Autodesk Fusion 360 part; units mm, degrees
note: some values were not read from the file. Chosen so that the rebuilt part matches the saved one: which bodies a step acts on; which face or edge a step refers to. Set by a fixed rule: which sketch regions a step uses.
(part 2 of 3)
  line L303 (277.1753, -95.3023) -> (279.6753, -95.3023)
  line L304 (279.6753, -95.3023) -> (279.6753, -95.8023)
  line L305 (279.6753, -95.8023) -> (277.1753, -95.8023)
  line L306 (274.6753, -80.803) -> (277.1753, -80.803)
  line L307 (279.6753, -80.803) -> (277.1753, -80.803)
  line L308 (279.6753, -81.303) -> (279.6753, -80.803)
  line L309 (274.6753, -81.303) -> (274.6753, -80.803)
  line L310 (277.1753, -81.303) -> (274.6753, -81.303)
  line L311 (277.1753, -81.303) -> (279.6753, -81.303)
  line L312 (260.6253, -95.8023) -> (258.1253, -95.8023)
  line L313 (255.6253, -95.8023) -> (258.1253, -95.8023)
  line L314 (255.6253, -95.3023) -> (255.6253, -95.8023)
  line L315 (260.6253, -95.3023) -> (260.6253, -95.8023)
  line L316 (258.1253, -95.3023) -> (260.6253, -95.3023)
  line L317 (258.1253, -95.3023) -> (255.6253, -95.3023)
  line L318 (258.1253, -81.303) -> (260.6253, -81.303)
  line L319 (260.6253, -81.303) -> (260.6253, -80.803)
  line L320 (260.6253, -80.803) -> (258.1253, -80.803)
  line L321 (255.6253, -80.803) -> (258.1253, -80.803)
  line L322 (255.6253, -81.303) -> (255.6253, -80.803)
  line L323 (258.1253, -81.303) -> (255.6253, -81.303)
  line L324 (239.0753, -81.303) -> (241.5753, -81.303)
  line L325 (236.5753, -80.803) -> (239.0753, -80.803)
  line L326 (236.5753, -81.303) -> (236.5753, -80.803)
  line L327 (241.5753, -95.8023) -> (239.0753, -95.8023)
  line L328 (239.0753, -81.303) -> (236.5753, -81.303)
  line L329 (239.0753, -95.3023) -> (236.5753, -95.3023)
  line L330 (236.5753, -95.3023) -> (236.5753, -95.8023)
  line L331 (241.5753, -81.303) -> (241.5753, -80.803)
  line L332 (241.5753, -80.803) -> (239.0753, -80.803)
  line L333 (241.5753, -95.3023) -> (241.5753, -95.8023)
  line L334 (236.5753, -95.8023) -> (239.0753, -95.8023)
  line L335 (239.0753, -95.3023) -> (241.5753, -95.3023)
  line L336 (217.5253, -95.3023) -> (217.5253, -95.8023)
  line L337 (217.5253, -80.803) -> (220.0253, -80.803)
  line L338 (222.5253, -95.3023) -> (222.5253, -95.8023)
  line L339 (220.0253, -81.303) -> (217.5253, -81.303)
  line L340 (217.5253, -81.303) -> (217.5253, -80.803)
  line L341 (217.5253, -95.8023) -> (220.0253, -95.8023)
  line L342 (220.0253, -95.3023) -> (222.5253, -95.3023)
  line L343 (220.0253, -95.3023) -> (217.5253, -95.3023)
  line L344 (222.5253, -80.803) -> (220.0253, -80.803)
  line L345 (222.5253, -81.303) -> (222.5253, -80.803)
  line L346 (220.0253, -81.303) -> (222.5253, -81.303)
  line L347 (222.5253, -95.8023) -> (220.0253, -95.8023)
  line L348 (198.4753, -95.3023) -> (198.4753, -95.8023)
  line L349 (198.4753, -80.803) -> (200.9753, -80.803)
  line L350 (203.4753, -95.3023) -> (203.4753, -95.8023)
  line L351 (200.9753, -81.303) -> (198.4753, -81.303)
  line L352 (198.4753, -81.303) -> (198.4753, -80.803)
  line L353 (198.4753, -95.8023) -> (200.9753, -95.8023)
  line L354 (200.9753, -95.3023) -> (203.4753, -95.3023)
  line L355 (200.9753, -95.3023) -> (198.4753, -95.3023)
  line L356 (203.4753, -80.803) -> (200.9753, -80.803)
  line L357 (203.4753, -81.303) -> (203.4753, -80.803)
  line L358 (200.9753, -81.303) -> (203.4753, -81.303)
  line L359 (203.4753, -95.8023) -> (200.9753, -95.8023)
  line L360 (179.4253, -95.8023) -> (181.9253, -95.8023)
  line L361 (184.4253, -95.3023) -> (184.4253, -95.8023)
  line L362 (179.4253, -95.3023) -> (179.4253, -95.8023)
  line L363 (181.9253, -95.3023) -> (184.4253, -95.3023)
  line L364 (181.9253, -95.3023) -> (179.4253, -95.3023)
  line L365 (184.4253, -95.8023) -> (181.9253, -95.8023)
  line L366 (179.4253, -81.303) -> (179.4253, -80.803)
  line L367 (179.4253, -80.803) -> (181.9253, -80.803)
  line L368 (184.4253, -81.303) -> (184.4253, -80.803)
  line L369 (181.9253, -81.303) -> (179.4253, -81.303)
  line L370 (181.9253, -81.303) -> (184.4253, -81.303)
  line L371 (184.4253, -80.803) -> (181.9253, -80.803)
  line L372 (160.3753, -95.8023) -> (162.8753, -95.8023)
  line L373 (165.3753, -95.8023) -> (162.8753, -95.8023)
  line L374 (162.8753, -95.3023) -> (165.3753, -95.3023)
  line L375 (165.3753, -95.3023) -> (165.3753, -95.8023)
  line L376 (160.3753, -95.3023) -> (160.3753, -95.8023)
  line L377 (162.8753, -95.3023) -> (160.3753, -95.3023)
  line L378 (160.3753, -81.303) -> (160.3753, -80.803)
  line L379 (165.3753, -81.303) -> (165.3753, -80.803)
  line L380 (162.8753, -81.303) -> (165.3753, -81.303)
  line L381 (160.3753, -80.803) -> (162.8753, -80.803)
  line L382 (165.3753, -80.803) -> (162.8753, -80.803)
  line L383 (162.8753, -81.303) -> (160.3753, -81.303)
  line L384 (141.3253, -95.8023) -> (143.8253, -95.8023)
  line L385 (143.8253, -95.3023) -> (146.3253, -95.3023)
  line L386 (141.3253, -95.3023) -> (141.3253, -95.8023)
  line L387 (146.3253, -95.8023) -> (143.8253, -95.8023)
  line L388 (143.8253, -95.3023) -> (141.3253, -95.3023)
  line L389 (146.3253, -95.3023) -> (146.3253, -95.8023)
  line L390 (141.3253, -81.303) -> (141.3253, -80.803)
  line L391 (143.8253, -81.303) -> (146.3253, -81.303)
  line L392 (143.8253, -81.303) -> (141.3253, -81.303)
  line L393 (146.3253, -81.303) -> (146.3253, -80.803)
  line L394 (141.3253, -80.803) -> (143.8253, -80.803)
  line L395 (146.3253, -80.803) -> (143.8253, -80.803)
  line L396 (122.2753, -95.3023) -> (122.2753, -95.8023)
  line L397 (124.7753, -95.3023) -> (127.2753, -95.3023)
  line L398 (122.2753, -95.8023) -> (124.7753, -95.8023)
  line L399 (124.7753, -95.3023) -> (122.2753, -95.3023)
  line L400 (127.2753, -95.3023) -> (127.2753, -95.8023)
  line L401 (127.2753, -95.8023) -> (124.7753, -95.8023)
  line L402 (122.2753, -81.303) -> (122.2753, -80.803)
  line L403 (127.2753, -81.303) -> (127.2753, -80.803)
  line L404 (122.2753, -80.803) -> (124.7753, -80.803)
  line L405 (124.7753, -81.303) -> (127.2753, -81.303)
  line L406 (124.7753, -81.303) -> (122.2753, -81.303)
  line L407 (127.2753, -80.803) -> (124.7753, -80.803)
  line L408 (108.2253, -95.3023) -> (108.2253, -95.8023)
  line L409 (108.2253, -95.8023) -> (105.7253, -95.8023)
  line L410 (105.7253, -95.3023) -> (103.2253, -95.3023)
  line L411 (103.2253, -95.8023) -> (105.7253, -95.8023)
  line L412 (105.7253, -95.3023) -> (108.2253, -95.3023)
  line L413 (103.2253, -95.3023) -> (103.2253, -95.8023)
  line L414 (103.2253, -80.803) -> (105.7253, -80.803)
  line L415 (105.7253, -81.303) -> (108.2253, -81.303)
  line L416 (108.2253, -80.803) -> (105.7253, -80.803)
  line L417 (105.7253, -81.303) -> (103.2253, -81.303)
  line L418 (108.2253, -81.303) -> (108.2253, -80.803)
  line L419 (103.2253, -81.303) -> (103.2253, -80.803)
  line L420 (89.1753, -95.3023) -> (89.1753, -95.8023)
  line L421 (84.1753, -95.3023) -> (84.1753, -95.8023)
  line L422 (86.6753, -95.3023) -> (89.1753, -95.3023)
  line L423 (84.1753, -95.8023) -> (86.6753, -95.8023)
  line L424 (86.6753, -95.3023) -> (84.1753, -95.3023)
  line L425 (89.1753, -95.8023) -> (86.6753, -95.8023)
  line L426 (89.1753, -81.303) -> (89.1753, -80.803)
  line L427 (86.6753, -81.303) -> (84.1753, -81.303)
  line L428 (84.1753, -81.303) -> (84.1753, -80.803)
  line L429 (84.1753, -80.803) -> (86.6753, -80.803)
  line L430 (89.1753, -80.803) -> (86.6753, -80.803)
  line L431 (86.6753, -81.303) -> (89.1753, -81.303)
  line L432 (70.1253, -95.3023) -> (70.1253, -95.8023)
  line L433 (67.6253, -95.3023) -> (65.1253, -95.3023)
  line L434 (65.1253, -95.8023) -> (67.6253, -95.8023)
  line L435 (67.6253, -95.3023) -> (70.1253, -95.3023)
  line L436 (65.1253, -95.3023) -> (65.1253, -95.8023)
  line L437 (70.1253, -95.8023) -> (67.6253, -95.8023)
  line L438 (65.1253, -80.803) -> (67.6253, -80.803)
  line L439 (70.1253, -80.803) -> (67.6253, -80.803)
  line L440 (67.6253, -81.303) -> (70.1253, -81.303)
  line L441 (65.1253, -81.303) -> (65.1253, -80.803)
  line L442 (70.1253, -81.303) -> (70.1253, -80.803)
  line L443 (67.6253, -81.303) -> (65.1253, -81.303)
  line L444 (51.0753, -95.8023) -> (48.5753, -95.8023)
  line L445 (51.0753, -95.3023) -> (51.0753, -95.8023)
  line L446 (48.5753, -95.3023) -> (46.0753, -95.3023)
  line L447 (46.0753, -95.3023) -> (46.0753, -95.8023)
  line L448 (48.5753, -95.3023) -> (51.0753, -95.3023)
  line L449 (46.0753, -95.8023) -> (48.5753, -95.8023)
  line L450 (46.0753, -81.303) -> (46.0753, -80.803)
  line L451 (48.5753, -81.303) -> (46.0753, -81.303)
  line L452 (48.5753, -81.303) -> (51.0753, -81.303)
  line L453 (51.0753, -80.803) -> (48.5753, -80.803)
  line L454 (51.0753, -81.303) -> (51.0753, -80.803)
  line L455 (46.0753, -80.803) -> (48.5753, -80.803)
  line L456 (32.0253, -95.8023) -> (29.5253, -95.8023)
  line L457 (27.0253, -95.3023) -> (27.0253, -95.8023)
  line L458 (29.5253, -95.3023) -> (32.0253, -95.3023)
  line L459 (29.5253, -95.3023) -> (27.0253, -95.3023)
  line L460 (32.0253, -95.3023) -> (32.0253, -95.8023)
  line L461 (27.0253, -95.8023) -> (29.5253, -95.8023)
  line L462 (32.0253, -81.303) -> (32.0253, -80.803)
  line L463 (27.0253, -81.303) -> (27.0253, -80.803)
  line L464 (27.0253, -80.803) -> (29.5253, -80.803)
  line L465 (32.0253, -80.803) -> (29.5253, -80.803)
  line L466 (29.5253, -81.303) -> (32.0253, -81.303)
  line L467 (29.5253, -81.303) -> (27.0253, -81.303)
  line L468 (10.4753, -95.3023) -> (7.9753, -95.3023)
  line L469 (7.9753, -95.8023) -> (10.4753, -95.8023)
  line L470 (12.9753, -95.3023) -> (12.9753, -95.8023)
  line L471 (12.9753, -95.8023) -> (10.4753, -95.8023)
  line L472 (7.9753, -95.3023) -> (7.9753, -95.8023)
  line L473 (10.4753, -95.3023) -> (12.9753, -95.3023)
  line L474 (12.9753, -80.803) -> (10.4753, -80.803)
  line L475 (10.4753, -81.303) -> (12.9753, -81.303)
  line L476 (7.9753, -81.303) -> (7.9753, -80.803)
  line L477 (10.4753, -81.303) -> (7.9753, -81.303)
  line L478 (12.9753, -81.303) -> (12.9753, -80.803)
  line L479 (7.9753, -80.803) -> (10.4753, -80.803)
  line L480 (296.2253, -76.2523) -> (298.7253, -76.2523)
  line L481 (298.7253, -76.2523) -> (298.7253, -76.7523)
  line L482 (298.7253, -76.7523) -> (296.2253, -76.7523)
  line L483 (296.2253, -76.2523) -> (293.7253, -76.2523)
  line L484 (293.7253, -76.2523) -> (293.7253, -76.7523)
  line L485 (293.7253, -76.7523) -> (296.2253, -76.7523)
  line L486 (274.9128, -76.2523) -> (274.9128, -76.7523)
  line L487 (272.4128, -76.2523) -> (269.9128, -76.2523)
  line L488 (269.9128, -76.7523) -> (272.4128, -76.7523)
  line L489 (274.9128, -76.7523) -> (272.4128, -76.7523)
  line L490 (272.4128, -76.2523) -> (274.9128, -76.2523)
  line L491 (269.9128, -76.2523) -> (269.9128, -76.7523)
  line L492 (251.1003, -76.7523) -> (248.6003, -76.7523)
  line L493 (248.6003, -76.2523) -> (246.1003, -76.2523)
  line L494 (246.1003, -76.2523) -> (246.1003, -76.7523)
  line L495 (251.1003, -76.2523) -> (251.1003, -76.7523)
  line L496 (248.6003, -76.2523) -> (251.1003, -76.2523)
  line L497 (246.1003, -76.7523) -> (248.6003, -76.7523)
  line L498 (227.0503, -76.2523) -> (227.0503, -76.7523)
  line L499 (229.5503, -76.2523) -> (232.0503, -76.2523)
  line L500 (232.0503, -76.2523) -> (232.0503, -76.7523)
  line L501 (227.0503, -76.7523) -> (229.5503, -76.7523)
  line L502 (232.0503, -76.7523) -> (229.5503, -76.7523)
  line L503 (229.5503, -76.2523) -> (227.0503, -76.2523)
  line L504 (210.5003, -76.2523) -> (208.0003, -76.2523)
  line L505 (208.0003, -76.7523) -> (210.5003, -76.7523)
  line L506 (213.0003, -76.7523) -> (210.5003, -76.7523)
  line L507 (213.0003, -76.2523) -> (213.0003, -76.7523)
  line L508 (208.0003, -76.2523) -> (208.0003, -76.7523)
  line L509 (210.5003, -76.2523) -> (213.0003, -76.2523)
  line L510 (191.4503, -76.2523) -> (188.9503, -76.2523)
  line L511 (193.9503, -76.2523) -> (193.9503, -76.7523)
  line L512 (193.9503, -76.7523) -> (191.4503, -76.7523)
  line L513 (191.4503, -76.2523) -> (193.9503, -76.2523)
  line L514 (188.9503, -76.2523) -> (188.9503, -76.7523)
  line L515 (188.9503, -76.7523) -> (191.4503, -76.7523)
  line L516 (169.9003, -76.7523) -> (172.4003, -76.7523)
  line L517 (172.4003, -76.2523) -> (174.9003, -76.2523)
  line L518 (174.9003, -76.7523) -> (172.4003, -76.7523)
  line L519 (172.4003, -76.2523) -> (169.9003, -76.2523)
  line L520 (169.9003, -76.2523) -> (169.9003, -76.7523)
  line L521 (174.9003, -76.2523) -> (174.9003, -76.7523)
  line L522 (153.3503, -76.2523) -> (150.8503, -76.2523)
  line L523 (155.8503, -76.2523) -> (155.8503, -76.7523)
  line L524 (150.8503, -76.2523) -> (150.8503, -76.7523)
  line L525 (155.8503, -76.7523) -> (153.3503, -76.7523)
  line L526 (153.3503, -76.2523) -> (155.8503, -76.2523)
  line L527 (150.8503, -76.7523) -> (153.3503, -76.7523)
  line L528 (134.3003, -76.2523) -> (131.8003, -76.2523)
  line L529 (131.8003, -76.2523) -> (131.8003, -76.7523)
  line L530 (136.8003, -76.2523) -> (136.8003, -76.7523)
  line L531 (131.8003, -76.7523) -> (134.3003, -76.7523)
  line L532 (136.8003, -76.7523) -> (134.3003, -76.7523)
  line L533 (134.3003, -76.2523) -> (136.8003, -76.2523)
  line L534 (117.7503, -76.7523) -> (115.2503, -76.7523)
  line L535 (112.7503, -76.2523) -> (112.7503, -76.7523)
  line L536 (115.2503, -76.2523) -> (117.7503, -76.2523)
  line L537 (117.7503, -76.2523) -> (117.7503, -76.7523)
  line L538 (115.2503, -76.2523) -> (112.7503, -76.2523)
  line L539 (112.7503, -76.7523) -> (115.2503, -76.7523)
  line L540 (93.7003, -76.7523) -> (96.2003, -76.7523)
  line L541 (93.7003, -76.2523) -> (93.7003, -76.7523)
  line L542 (98.7003, -76.7523) -> (96.2003, -76.7523)
  line L543 (98.7003, -76.2523) -> (98.7003, -76.7523)
  line L544 (96.2003, -76.2523) -> (93.7003, -76.2523)
  line L545 (96.2003, -76.2523) -> (98.7003, -76.2523)
  line L546 (77.1503, -76.2523) -> (79.6503, -76.2523)
  line L547 (79.6503, -76.2523) -> (79.6503, -76.7523)
  line L548 (77.1503, -76.2523) -> (74.6503, -76.2523)
  line L549 (79.6503, -76.7523) -> (77.1503, -76.7523)
  line L550 (74.6503, -76.7523) -> (77.1503, -76.7523)
  line L551 (74.6503, -76.2523) -> (74.6503, -76.7523)
  line L552 (58.1003, -76.2523) -> (60.6003, -76.2523)
  line L553 (60.6003, -76.7523) -> (58.1003, -76.7523)
  line L554 (55.6003, -76.7523) -> (58.1003, -76.7523)
  line L555 (60.6003, -76.2523) -> (60.6003, -76.7523)
  line L556 (58.1003, -76.2523) -> (55.6003, -76.2523)
  line L557 (55.6003, -76.2523) -> (55.6003, -76.7523)
  line L558 (41.5503, -76.7523) -> (39.0503, -76.7523)
  line L559 (36.5503, -76.2523) -> (36.5503, -76.7523)
  line L560 (41.5503, -76.2523) -> (41.5503, -76.7523)
  line L561 (36.5503, -76.7523) -> (39.0503, -76.7523)
  line L562 (39.0503, -76.2523) -> (36.5503, -76.2523)
  line L563 (39.0503, -76.2523) -> (41.5503, -76.2523)
  line L564 (15.2378, -76.2523) -> (17.7378, -76.2523)
  line L565 (17.7378, -76.7523) -> (15.2378, -76.7523)
  line L566 (12.7378, -76.2523) -> (12.7378, -76.7523)
  line L567 (12.7378, -76.7523) -> (15.2378, -76.7523)
  line L568 (15.2378, -76.2523) -> (12.7378, -76.2523)
  line L569 (17.7378, -76.2523) -> (17.7378, -76.7523)
  line L570 (298.7253, -62.253) -> (298.7253, -61.753)
  line L571 (293.7253, -61.753) -> (296.2253, -61.753)
  line L572 (296.2253, -62.253) -> (298.7253, -62.253)
  line L573 (296.2253, -62.253) -> (293.7253, -62.253)
  line L574 (293.7253, -62.253) -> (293.7253, -61.753)
  line L575 (298.7253, -61.753) -> (296.2253, -61.753)
  line L576 (274.9128, -61.753) -> (272.4128, -61.753)
  line L577 (272.4128, -62.253) -> (269.9128, -62.253)
  line L578 (269.9128, -62.253) -> (269.9128, -61.753)
  line L579 (269.9128, -61.753) -> (272.4128, -61.753)
  line L580 (272.4128, -62.253) -> (274.9128, -62.253)
  line L581 (274.9128, -62.253) -> (274.9128, -61.753)
  line L582 (251.1003, -62.253) -> (251.1003, -61.753)
  line L583 (246.1003, -61.753) -> (248.6003, -61.753)
  line L584 (246.1003, -62.253) -> (246.1003, -61.753)
  line L585 (248.6003, -62.253) -> (251.1003, -62.253)
  line L586 (248.6003, -62.253) -> (246.1003, -62.253)
  line L587 (251.1003, -61.753) -> (248.6003, -61.753)
  line L588 (229.5503, -62.253) -> (232.0503, -62.253)
  line L589 (232.0503, -62.253) -> (232.0503, -61.753)
  line L590 (232.0503, -61.753) -> (229.5503, -61.753)
  line L591 (227.0503, -61.753) -> (229.5503, -61.753)
  line L592 (229.5503, -62.253) -> (227.0503, -62.253)
  line L593 (227.0503, -62.253) -> (227.0503, -61.753)
  line L594 (208.0003, -61.753) -> (210.5003, -61.753)
  line L595 (210.5003, -62.253) -> (213.0003, -62.253)
  line L596 (213.0003, -61.753) -> (210.5003, -61.753)
  line L597 (208.0003, -62.253) -> (208.0003, -61.753)
  line L598 (213.0003, -62.253) -> (213.0003, -61.753)
  line L599 (210.5003, -62.253) -> (208.0003, -62.253)
  line L600 (188.9503, -62.253) -> (188.9503, -61.753)
  line L601 (188.9503, -61.753) -> (191.4503, -61.753)
  line L602 (191.4503, -62.253) -> (188.9503, -62.253)
  line L603 (191.4503, -62.253) -> (193.9503, -62.253)
  line L604 (193.9503, -61.753) -> (191.4503, -61.753)
  line L605 (193.9503, -62.253) -> (193.9503, -61.753)
  line L606 (174.9003, -62.253) -> (174.9003, -61.753)
  line L607 (174.9003, -61.753) -> (172.4003, -61.753)
  line L608 (172.4003, -62.253) -> (174.9003, -62.253)
  line L609 (169.9003, -61.753) -> (172.4003, -61.753)
  line L610 (172.4003, -62.253) -> (169.9003, -62.253)
  line L611 (169.9003, -62.253) -> (169.9003, -61.753)
  line L612 (153.3503, -62.253) -> (155.8503, -62.253)
  line L613 (155.8503, -62.253) -> (155.8503, -61.753)
  line L614 (153.3503, -62.253) -> (150.8503, -62.253)
  line L615 (155.8503, -61.753) -> (153.3503, -61.753)
  line L616 (150.8503, -61.753) -> (153.3503, -61.753)
  line L617 (150.8503, -62.253) -> (150.8503, -61.753)
  line L618 (134.3003, -62.253) -> (131.8003, -62.253)
  line L619 (134.3003, -62.253) -> (136.8003, -62.253)
  line L620 (131.8003, -61.753) -> (134.3003, -61.753)
  line L621 (136.8003, -62.253) -> (136.8003, -61.753)
  line L622 (136.8003, -61.753) -> (134.3003, -61.753)
  line L623 (131.8003, -62.253) -> (131.8003, -61.753)
  line L624 (117.7503, -61.753) -> (115.2503, -61.753)
  line L625 (112.7503, -62.253) -> (112.7503, -61.753)
  line L626 (112.7503, -61.753) -> (115.2503, -61.753)
  line L627 (115.2503, -62.253) -> (117.7503, -62.253)
  line L628 (117.7503, -62.253) -> (117.7503, -61.753)
  line L629 (115.2503, -62.253) -> (112.7503, -62.253)
  line L630 (98.7003, -61.753) -> (96.2003, -61.753)
  line L631 (96.2003, -62.253) -> (93.7003, -62.253)
  line L632 (93.7003, -61.753) -> (96.2003, -61.753)
  line L633 (93.7003, -62.253) -> (93.7003, -61.753)
  line L634 (96.2003, -62.253) -> (98.7003, -62.253)
  line L635 (98.7003, -62.253) -> (98.7003, -61.753)
  line L636 (77.1503, -62.253) -> (79.6503, -62.253)
  line L637 (74.6503, -62.253) -> (74.6503, -61.753)
  line L638 (77.1503, -62.253) -> (74.6503, -62.253)
  line L639 (79.6503, -61.753) -> (77.1503, -61.753)
  line L640 (74.6503, -61.753) -> (77.1503, -61.753)
  line L641 (79.6503, -62.253) -> (79.6503, -61.753)
  line L642 (55.6003, -61.753) -> (58.1003, -61.753)
  line L643 (58.1003, -62.253) -> (55.6003, -62.253)
  line L644 (60.6003, -62.253) -> (60.6003, -61.753)
  line L645 (55.6003, -62.253) -> (55.6003, -61.753)
  line L646 (58.1003, -62.253) -> (60.6003, -62.253)
  line L647 (60.6003, -61.753) -> (58.1003, -61.753)
  line L648 (39.0503, -62.253) -> (41.5503, -62.253)
  line L649 (39.0503, -62.253) -> (36.5503, -62.253)
  line L650 (36.5503, -61.753) -> (39.0503, -61.753)
  line L651 (41.5503, -62.253) -> (41.5503, -61.753)
  line L652 (41.5503, -61.753) -> (39.0503, -61.753)
  line L653 (36.5503, -62.253) -> (36.5503, -61.753)
  line L654 (17.7378, -62.253) -> (17.7378, -61.753)
  line L655 (17.7378, -61.753) -> (15.2378, -61.753)
  line L656 (12.7378, -61.753) -> (15.2378, -61.753)
  line L657 (15.2378, -62.253) -> (17.7378, -62.253)
  line L658 (15.2378, -62.253) -> (12.7378, -62.253)
  line L659 (12.7378, -62.253) -> (12.7378, -61.753)
  line L660 (296.2253, -43.203) -> (293.7253, -43.203)
  line L661 (293.7253, -42.703) -> (296.2253, -42.703)
  line L662 (293.7253, -43.203) -> (293.7253, -42.703)
  line L663 (298.7253, -42.703) -> (296.2253, -42.703)
  line L664 (298.7253, -43.203) -> (298.7253, -42.703)
  line L665 (296.2253, -43.203) -> (298.7253, -43.203)
  line L666 (296.2253, -57.2023) -> (293.7253, -57.2023)
  line L667 (296.2253, -57.2023) -> (298.7253, -57.2023)
  line L668 (298.7253, -57.2023) -> (298.7253, -57.7023)
  line L669 (293.7253, -57.2023) -> (293.7253, -57.7023)
  line L670 (293.7253, -57.7023) -> (296.2253, -57.7023)
  line L671 (298.7253, -57.7023) -> (296.2253, -57.7023)
  line L672 (265.2683, -57.2023) -> (262.7683, -57.2023)
  line L673 (262.7683, -57.2023) -> (262.7683, -57.7023)
  line L674 (262.7683, -57.7023) -> (265.2683, -57.7023)
  line L675 (265.2683, -57.2023) -> (267.7683, -57.2023)
  line L676 (267.7683, -57.2023) -> (267.7683, -57.7023)
  line L677 (267.7683, -57.7023) -> (265.2683, -57.7023)
  line L678 (265.2683, -43.203) -> (262.7683, -43.203)
  line L679 (265.2683, -43.203) -> (267.7683, -43.203)
  line L680 (262.7683, -43.203) -> (262.7683, -42.703)
  line L681 (267.7683, -42.703) -> (265.2683, -42.703)
  line L682 (267.7683, -43.203) -> (267.7683, -42.703)
  line L683 (262.7683, -42.703) -> (265.2683, -42.703)
  line L684 (234.3128, -57.2023) -> (231.8128, -57.2023)
  line L685 (231.8128, -57.2023) -> (231.8128, -57.7023)
  line L686 (231.8128, -57.7023) -> (234.3128, -57.7023)
  line L687 (234.3128, -57.2023) -> (236.8128, -57.2023)
  line L688 (236.8128, -57.2023) -> (236.8128, -57.7023)
  line L689 (236.8128, -57.7023) -> (234.3128, -57.7023)
  line L690 (234.3128, -43.203) -> (236.8128, -43.203)
  line L691 (231.8128, -42.703) -> (234.3128, -42.703)
  line L692 (236.8128, -42.703) -> (234.3128, -42.703)
  line L693 (236.8128, -43.203) -> (236.8128, -42.703)
  line L694 (231.8128, -43.203) -> (231.8128, -42.703)
  line L695 (234.3128, -43.203) -> (231.8128, -43.203)
  line L696 (217.7628, -57.7023) -> (215.2628, -57.7023)
  line L697 (215.2628, -57.2023) -> (217.7628, -57.2023)
  line L698 (215.2628, -43.203) -> (217.7628, -43.203)
  line L699 (217.7628, -42.703) -> (215.2628, -42.703)
  line L700 (212.7628, -42.703) -> (215.2628, -42.703)
  line L701 (215.2628, -57.2023) -> (212.7628, -57.2023)
  line L702 (212.7628, -57.2023) -> (212.7628, -57.7023)
  line L703 (212.7628, -43.203) -> (212.7628, -42.703)
  line L704 (217.7628, -57.2023) -> (217.7628, -57.7023)
  line L705 (212.7628, -57.7023) -> (215.2628, -57.7023)
  line L706 (215.2628, -43.203) -> (212.7628, -43.203)
  line L707 (217.7628, -43.203) -> (217.7628, -42.703)
  line L708 (196.2128, -43.203) -> (193.7128, -43.203)
  line L709 (196.2128, -57.2023) -> (193.7128, -57.2023)
  line L710 (193.7128, -57.2023) -> (193.7128, -57.7023)
  line L711 (193.7128, -42.703) -> (196.2128, -42.703)
  line L712 (198.7128, -42.703) -> (196.2128, -42.703)
  line L713 (196.2128, -57.2023) -> (198.7128, -57.2023)
  line L714 (198.7128, -57.7023) -> (196.2128, -57.7023)
  line L715 (198.7128, -43.203) -> (198.7128, -42.703)
  line L716 (196.2128, -43.203) -> (198.7128, -43.203)
  line L717 (198.7128, -57.2023) -> (198.7128, -57.7023)
  line L718 (193.7128, -57.7023) -> (196.2128, -57.7023)
  line L719 (193.7128, -43.203) -> (193.7128, -42.703)
  line L720 (177.1628, -43.203) -> (174.6628, -43.203)
  line L721 (179.6628, -57.2023) -> (179.6628, -57.7023)
  line L722 (174.6628, -57.7023) -> (177.1628, -57.7023)
  line L723 (179.6628, -42.703) -> (177.1628, -42.703)
  line L724 (177.1628, -43.203) -> (179.6628, -43.203)
  line L725 (177.1628, -57.2023) -> (174.6628, -57.2023)
  line L726 (174.6628, -57.2023) -> (174.6628, -57.7023)
  line L727 (174.6628, -42.703) -> (177.1628, -42.703)
  line L728 (179.6628, -57.7023) -> (177.1628, -57.7023)
  line L729 (174.6628, -43.203) -> (174.6628, -42.703)
  line L730 (179.6628, -43.203) -> (179.6628, -42.703)
  line L731 (177.1628, -57.2023) -> (179.6628, -57.2023)
  line L732 (158.1128, -57.2023) -> (155.6128, -57.2023)
  line L733 (160.6128, -57.7023) -> (158.1128, -57.7023)
  line L734 (160.6128, -42.703) -> (158.1128, -42.703)
  line L735 (158.1128, -43.203) -> (160.6128, -43.203)
  line L736 (158.1128, -57.2023) -> (160.6128, -57.2023)
  line L737 (160.6128, -43.203) -> (160.6128, -42.703)
  line L738 (160.6128, -57.2023) -> (160.6128, -57.7023)
  line L739 (155.6128, -42.703) -> (158.1128, -42.703)
  line L740 (155.6128, -57.7023) -> (158.1128, -57.7023)
  line L741 (155.6128, -57.2023) -> (155.6128, -57.7023)
  line L742 (155.6128, -43.203) -> (155.6128, -42.703)
  line L743 (158.1128, -43.203) -> (155.6128, -43.203)
  line L744 (136.5628, -43.203) -> (136.5628, -42.703)
  line L745 (136.5628, -57.7023) -> (139.0628, -57.7023)
  line L746 (136.5628, -42.703) -> (139.0628, -42.703)
  line L747 (141.5628, -42.703) -> (139.0628, -42.703)
  line L748 (139.0628, -57.2023) -> (136.5628, -57.2023)
  line L749 (141.5628, -57.7023) -> (139.0628, -57.7023)
  line L750 (141.5628, -57.2023) -> (141.5628, -57.7023)
  line L751 (139.0628, -57.2023) -> (141.5628, -57.2023)
  line L752 (136.5628, -57.2023) -> (136.5628, -57.7023)
  line L753 (139.0628, -43.203) -> (141.5628, -43.203)
  line L754 (139.0628, -43.203) -> (136.5628, -43.203)
  line L755 (141.5628, -43.203) -> (141.5628, -42.703)
  line L756 (120.0128, -57.2023) -> (117.5128, -57.2023)
  line L757 (117.5128, -57.7023) -> (120.0128, -57.7023)
  line L758 (117.5128, -57.2023) -> (117.5128, -57.7023)
  line L759 (117.5128, -42.703) -> (120.0128, -42.703)
  line L760 (117.5128, -43.203) -> (117.5128, -42.703)
  line L761 (120.0128, -57.2023) -> (122.5128, -57.2023)
  line L762 (120.0128, -43.203) -> (122.5128, -43.203)
  line L763 (122.5128, -57.7023) -> (120.0128, -57.7023)
  line L764 (122.5128, -57.2023) -> (122.5128, -57.7023)
  line L765 (122.5128, -43.203) -> (122.5128, -42.703)
  line L766 (120.0128, -43.203) -> (117.5128, -43.203)
  line L767 (122.5128, -42.703) -> (120.0128, -42.703)
  line L768 (100.9628, -57.2023) -> (103.4628, -57.2023)
  line L769 (103.4628, -57.7023) -> (100.9628, -57.7023)
  line L770 (103.4628, -42.703) -> (100.9628, -42.703)
  line L771 (103.4628, -43.203) -> (103.4628, -42.703)
  line L772 (100.9628, -43.203) -> (103.4628, -43.203)
  line L773 (98.4628, -42.703) -> (100.9628, -42.703)
  line L774 (103.4628, -57.2023) -> (103.4628, -57.7023)
  line L775 (98.4628, -57.7023) -> (100.9628, -57.7023)
  line L776 (100.9628, -57.2023) -> (98.4628, -57.2023)
  line L777 (98.4628, -43.203) -> (98.4628, -42.703)
  line L778 (98.4628, -57.2023) -> (98.4628, -57.7023)
  line L779 (100.9628, -43.203) -> (98.4628, -43.203)
  line L780 (79.4128, -42.703) -> (81.9128, -42.703)
  line L781 (84.4128, -42.703) -> (81.9128, -42.703)
  line L782 (81.9128, -57.2023) -> (79.4128, -57.2023)
  line L783 (79.4128, -57.7023) -> (81.9128, -57.7023)
  line L784 (79.4128, -43.203) -> (79.4128, -42.703)
  line L785 (81.9128, -43.203) -> (84.4128, -43.203)
  line L786 (84.4128, -43.203) -> (84.4128, -42.703)
  line L787 (84.4128, -57.2023) -> (84.4128, -57.7023)
  line L788 (81.9128, -57.2023) -> (84.4128, -57.2023)
  line L789 (79.4128, -57.2023) -> (79.4128, -57.7023)
  line L790 (81.9128, -43.203) -> (79.4128, -43.203)
  line L791 (84.4128, -57.7023) -> (81.9128, -57.7023)
  line L792 (62.8628, -57.2023) -> (60.3628, -57.2023)
  line L793 (65.3628, -57.7023) -> (62.8628, -57.7023)
  line L794 (62.8628, -43.203) -> (60.3628, -43.203)
  line L795 (62.8628, -57.2023) -> (65.3628, -57.2023)
  line L796 (60.3628, -57.7023) -> (62.8628, -57.7023)
  line L797 (65.3628, -42.703) -> (62.8628, -42.703)
  line L798 (62.8628, -43.203) -> (65.3628, -43.203)
  line L799 (60.3628, -42.703) -> (62.8628, -42.703)
  line L800 (65.3628, -43.203) -> (65.3628, -42.703)
  line L801 (60.3628, -57.2023) -> (60.3628, -57.7023)
  line L802 (60.3628, -43.203) -> (60.3628, -42.703)
  line L803 (65.3628, -57.2023) -> (65.3628, -57.7023)
  line L804 (41.3128, -42.703) -> (43.8128, -42.703)
  line L805 (43.8128, -43.203) -> (41.3128, -43.203)
  line L806 (46.3128, -43.203) -> (46.3128, -42.703)
  line L807 (46.3128, -57.2023) -> (46.3128, -57.7023)
  line L808 (41.3128, -43.203) -> (41.3128, -42.703)
  line L809 (43.8128, -57.2023) -> (46.3128, -57.2023)
  line L810 (41.3128, -57.7023) -> (43.8128, -57.7023)
  line L811 (41.3128, -57.2023) -> (41.3128, -57.7023)
  line L812 (46.3128, -57.7023) -> (43.8128, -57.7023)
  line L813 (43.8128, -57.2023) -> (41.3128, -57.2023)
  line L814 (46.3128, -42.703) -> (43.8128, -42.703)
  line L815 (43.8128, -43.203) -> (46.3128, -43.203)
  line L816 (17.6182, -57.2023) -> (15.1182, -57.2023)
  line L817 (15.1182, -57.2023) -> (15.1182, -57.7023)
  line L818 (15.1182, -57.7023) -> (17.6182, -57.7023)
  line L819 (17.6182, -57.2023) -> (20.1182, -57.2023)
  line L820 (20.1182, -57.2023) -> (20.1182, -57.7023)
  line L821 (20.1182, -57.7023) -> (17.6182, -57.7023)
  line L822 (20.1182, -42.703) -> (17.6182, -42.703)
  line L823 (17.6182, -43.203) -> (15.1182, -43.203)
  line L824 (17.6182, -43.203) -> (20.1182, -43.203)
  line L825 (15.1182, -42.703) -> (17.6182, -42.703)
  line L826 (15.1182, -43.203) -> (15.1182, -42.703)
  line L827 (20.1182, -43.203) -> (20.1182, -42.703)
  line L828 (293.7253, -24.1529) -> (293.7253, -23.6529)
  line L829 (293.7253, -23.6529) -> (296.2253, -23.6529)
  line L830 (296.2253, -24.1529) -> (298.7253, -24.1529)
  line L831 (298.7253, -24.1529) -> (298.7253, -23.6529)
  line L832 (296.2253, -24.1529) -> (293.7253, -24.1529)
  line L833 (293.7253, -38.6522) -> (296.2253, -38.6522)
  line L834 (296.2253, -38.1522) -> (298.7253, -38.1522)
  line L835 (296.2253, -38.1522) -> (293.7253, -38.1522)
  line L836 (298.7253, -38.6522) -> (296.2253, -38.6522)
  line L837 (298.7253, -38.1522) -> (298.7253, -38.6522)
  line L838 (298.7253, -23.6529) -> (296.2253, -23.6529)
  line L839 (293.7253, -38.1522) -> (293.7253, -38.6522)
  line L840 (279.6753, -24.1529) -> (279.6753, -23.6529)
  line L841 (279.6753, -38.6522) -> (277.1753, -38.6522)
  line L842 (274.6753, -24.1529) -> (274.6753, -23.6529)
  line L843 (277.1753, -24.1529) -> (279.6753, -24.1529)
  line L844 (274.6753, -38.1522) -> (274.6753, -38.6522)
  line L845 (274.6753, -23.6529) -> (277.1753, -23.6529)
  line L846 (277.1753, -24.1529) -> (274.6753, -24.1529)
  line L847 (274.6753, -38.6522) -> (277.1753, -38.6522)
  line L848 (279.6753, -23.6529) -> (277.1753, -23.6529)
  line L849 (279.6753, -38.1522) -> (279.6753, -38.6522)
  line L850 (277.1753, -38.1522) -> (274.6753, -38.1522)
  line L851 (277.1753, -38.1522) -> (279.6753, -38.1522)
  line L852 (296.2253, -5.1029) -> (293.7253, -5.1029)
  line L853 (293.7253, -19.1022) -> (293.7253, -19.6022)
  line L854 (293.7253, -5.1029) -> (293.7253, -4.6029)
  line L855 (296.2253, -5.1029) -> (298.7253, -5.1029)
  line L856 (296.2253, -19.1022) -> (293.7253, -19.1022)
  line L857 (298.7253, -4.6029) -> (296.2253, -4.6029)
  line L858 (293.7253, -4.6029) -> (296.2253, -4.6029)
  line L859 (298.7253, -19.1022) -> (298.7253, -19.6022)
  line L860 (296.2253, -19.1022) -> (298.7253, -19.1022)
  line L861 (298.7253, -19.6022) -> (296.2253, -19.6022)
  line L862 (298.7253, -5.1029) -> (298.7253, -4.6029)
  line L863 (293.7253, -19.6022) -> (296.2253, -19.6022)
  line L864 (277.1753, -5.1029) -> (279.6753, -5.1029)
  line L865 (274.6753, -19.6022) -> (277.1753, -19.6022)
  line L866 (274.6753, -5.1029) -> (274.6753, -4.6029)
  line L867 (274.6753, -19.1022) -> (274.6753, -19.6022)
  line L868 (274.6753, -4.6029) -> (277.1753, -4.6029)
  line L869 (277.1753, -19.1022) -> (274.6753, -19.1022)
  line L870 (279.6753, -4.6029) -> (277.1753, -4.6029)
  line L871 (279.6753, -5.1029) -> (279.6753, -4.6029)
  line L872 (277.1753, -19.1022) -> (279.6753, -19.1022)
  line L873 (279.6753, -19.6022) -> (277.1753, -19.6022)
  line L874 (277.1753, -5.1029) -> (274.6753, -5.1029)
  line L875 (279.6753, -19.1022) -> (279.6753, -19.6022)
  line L876 (224.7878, -38.1522) -> (222.2878, -38.1522)
  line L877 (222.2878, -38.1522) -> (222.2878, -38.6522)
  line L878 (222.2878, -38.6522) -> (224.7878, -38.6522)
  line L879 (224.7878, -38.1522) -> (227.2878, -38.1522)
  line L880 (227.2878, -38.1522) -> (227.2878, -38.6522)
  line L881 (227.2878, -38.6522) -> (224.7878, -38.6522)
  line L882 (227.2878, -23.6528) -> (224.7878, -23.6528)
  line L883 (222.2878, -24.1528) -> (222.2878, -23.6528)
  line L884 (224.7878, -24.1528) -> (222.2878, -24.1528)
  line L885 (222.2878, -23.6528) -> (224.7878, -23.6528)
  line L886 (224.7878, -24.1528) -> (227.2878, -24.1528)
  line L887 (227.2878, -24.1528) -> (227.2878, -23.6528)
  line L888 (208.2378, -38.6522) -> (205.7378, -38.6522)
  line L889 (205.7378, -24.1528) -> (203.2378, -24.1528)
  line L890 (203.2378, -23.6528) -> (205.7378, -23.6528)
  line L891 (208.2378, -38.1522) -> (208.2378, -38.6522)
  line L892 (208.2378, -24.1528) -> (208.2378, -23.6528)
  line L893 (205.7378, -38.1522) -> (208.2378, -38.1522)
  line L894 (205.7378, -24.1528) -> (208.2378, -24.1528)
  line L895 (203.2378, -38.1522) -> (203.2378, -38.6522)
  line L896 (203.2378, -24.1528) -> (203.2378, -23.6528)
  line L897 (208.2378, -23.6528) -> (205.7378, -23.6528)
  line L898 (205.7378, -38.1522) -> (203.2378, -38.1522)
  line L899 (203.2378, -38.6522) -> (205.7378, -38.6522)
  line L900 (189.1878, -38.1522) -> (189.1878, -38.6522)
  line L901 (189.1878, -23.6528) -> (186.6878, -23.6528)
  line L902 (184.1878, -23.6528) -> (186.6878, -23.6528)
  line L903 (186.6878, -38.1522) -> (189.1878, -38.1522)
  line L904 (184.1878, -38.1522) -> (184.1878, -38.6522)
  line L905 (186.6878, -24.1528) -> (189.1878, -24.1528)
  line L906 (189.1878, -38.6522) -> (186.6878, -38.6522)
  line L907 (186.6878, -38.1522) -> (184.1878, -38.1522)
  line L908 (184.1878, -24.1528) -> (184.1878, -23.6528)
  line L909 (189.1878, -24.1528) -> (189.1878, -23.6528)
  line L910 (184.1878, -38.6522) -> (186.6878, -38.6522)
  line L911 (186.6878, -24.1528) -> (184.1878, -24.1528)
  line L912 (167.6378, -24.1528) -> (170.1378, -24.1528)
  line L913 (167.6378, -24.1528) -> (165.1378, -24.1528)
  line L914 (170.1378, -24.1528) -> (170.1378, -23.6528)
  line L915 (170.1378, -23.6528) -> (167.6378, -23.6528)
  line L916 (170.1378, -38.1522) -> (170.1378, -38.6522)
  line L917 (170.1378, -38.6522) -> (167.6378, -38.6522)
  line L918 (165.1378, -38.6522) -> (167.6378, -38.6522)
  line L919 (165.1378, -23.6528) -> (167.6378, -23.6528)
  line L920 (165.1378, -24.1528) -> (165.1378, -23.6528)
  line L921 (165.1378, -38.1522) -> (165.1378, -38.6522)
  line L922 (167.6378, -38.1522) -> (170.1378, -38.1522)
  line L923 (167.6378, -38.1522) -> (165.1378, -38.1522)
  line L924 (88.9378, -38.1522) -> (88.9378, -38.6522)
  line L925 (93.9378, -23.6528) -> (91.4378, -23.6528)
  line L926 (88.9378, -23.6528) -> (91.4378, -23.6528)
  line L927 (91.4378, -24.1528) -> (88.9378, -24.1528)
  line L928 (91.4378, -24.1528) -> (93.9378, -24.1528)
  line L929 (91.4378, -38.1522) -> (93.9378, -38.1522)
  line L930 (88.9378, -38.6522) -> (91.4378, -38.6522)
  line L931 (88.9378, -24.1528) -> (88.9378, -23.6528)
  line L932 (91.4378, -38.1522) -> (88.9378, -38.1522)
  line L933 (93.9378, -38.6522) -> (91.4378, -38.6522)
  line L934 (93.9378, -24.1528) -> (93.9378, -23.6528)
  line L935 (93.9378, -38.1522) -> (93.9378, -38.6522)
  line L936 (112.9878, -38.1522) -> (112.9878, -38.6522)
  line L937 (107.9878, -24.1528) -> (107.9878, -23.6528)
  line L938 (107.9878, -23.6528) -> (110.4878, -23.6528)
  line L939 (110.4878, -24.1528) -> (107.9878, -24.1528)
  line L940 (110.4878, -38.1522) -> (107.9878, -38.1522)
  line L941 (107.9878, -38.6522) -> (110.4878, -38.6522)
  line L942 (112.9878, -38.6522) -> (110.4878, -38.6522)
  line L943 (110.4878, -38.1522) -> (112.9878, -38.1522)
  line L944 (110.4878, -24.1528) -> (112.9878, -24.1528)
  line L945 (107.9878, -38.1522) -> (107.9878, -38.6522)
  line L946 (112.9878, -24.1528) -> (112.9878, -23.6528)
  line L947 (112.9878, -23.6528) -> (110.4878, -23.6528)
  line L948 (132.0378, -38.1522) -> (132.0378, -38.6522)
  line L949 (132.0378, -38.6522) -> (129.5378, -38.6522)
  line L950 (127.0378, -38.6522) -> (129.5378, -38.6522)
  line L951 (127.0378, -38.1522) -> (127.0378, -38.6522)
  line L952 (129.5378, -24.1528) -> (127.0378, -24.1528)
  line L953 (129.5378, -24.1528) -> (132.0378, -24.1528)
  line L954 (127.0378, -24.1528) -> (127.0378, -23.6528)
  line L955 (129.5378, -38.1522) -> (127.0378, -38.1522)
  line L956 (129.5378, -38.1522) -> (132.0378, -38.1522)
  line L957 (132.0378, -24.1528) -> (132.0378, -23.6528)
  line L958 (132.0378, -23.6528) -> (129.5378, -23.6528)
  line L959 (127.0378, -23.6528) -> (129.5378, -23.6528)
  line L960 (148.5878, -38.1522) -> (146.0878, -38.1522)
  line L961 (148.5878, -24.1528) -> (146.0878, -24.1528)
  line L962 (146.0878, -24.1528) -> (146.0878, -23.6528)
  line L963 (151.0878, -24.1528) -> (151.0878, -23.6528)
  line L964 (146.0878, -38.6522) -> (148.5878, -38.6522)
  line L965 (151.0878, -38.1522) -> (151.0878, -38.6522)
  line L966 (151.0878, -23.6528) -> (148.5878, -23.6528)
  line L967 (148.5878, -38.1522) -> (151.0878, -38.1522)
  line L968 (146.0878, -23.6528) -> (148.5878, -23.6528)
  line L969 (151.0878, -38.6522) -> (148.5878, -38.6522)
  line L970 (148.5878, -24.1528) -> (151.0878, -24.1528)
  line L971 (146.0878, -38.1522) -> (146.0878, -38.6522)
  line L972 (53.3378, -38.1522) -> (50.8378, -38.1522)
  line L973 (55.8378, -23.6528) -> (53.3378, -23.6528)
  line L974 (50.8378, -23.6528) -> (53.3378, -23.6528)
  line L975 (53.3378, -24.1528) -> (50.8378, -24.1528)
  line L976 (55.8378, -24.1528) -> (55.8378, -23.6528)
  line L977 (53.3378, -24.1528) -> (55.8378, -24.1528)
  line L978 (55.8378, -38.1522) -> (55.8378, -38.6522)
  line L979 (50.8378, -38.1522) -> (50.8378, -38.6522)
  line L980 (50.8378, -38.6522) -> (53.3378, -38.6522)
  line L981 (55.8378, -38.6522) -> (53.3378, -38.6522)
  line L982 (50.8378, -24.1528) -> (50.8378, -23.6528)
  line L983 (53.3378, -38.1522) -> (55.8378, -38.1522)
  line L984 (74.8878, -24.1528) -> (74.8878, -23.6528)
  line L985 (72.3878, -38.1522) -> (74.8878, -38.1522)
  line L986 (69.8878, -23.6528) -> (72.3878, -23.6528)
  line L987 (69.8878, -38.1522) -> (69.8878, -38.6522)
  line L988 (74.8878, -38.6522) -> (72.3878, -38.6522)
  line L989 (69.8878, -24.1528) -> (69.8878, -23.6528)
  line L990 (72.3878, -38.1522) -> (69.8878, -38.1522)
  line L991 (74.8878, -38.1522) -> (74.8878, -38.6522)
  line L992 (69.8878, -38.6522) -> (72.3878, -38.6522)
  line L993 (74.8878, -23.6528) -> (72.3878, -23.6528)
  line L994 (72.3878, -24.1528) -> (74.8878, -24.1528)
  line L995 (72.3878, -24.1528) -> (69.8878, -24.1528)
  line L996 (22.3814, -38.1522) -> (19.8814, -38.1522)
  line L997 (19.8814, -38.1522) -> (19.8814, -38.6522)
  line L998 (19.8814, -38.6522) -> (22.3814, -38.6522)
  line L999 (22.3814, -38.1522) -> (24.8814, -38.1522)
  line L1000 (24.8814, -38.1522) -> (24.8814, -38.6522)
  line L1001 (24.8814, -38.6522) -> (22.3814, -38.6522)
  line L1002 (19.8814, -23.6528) -> (22.3814, -23.6528)
  line L1003 (19.8814, -24.1528) -> (19.8814, -23.6528)
  line L1004 (24.8814, -24.1528) -> (24.8814, -23.6528)
  line L1005 (22.3814, -24.1528) -> (19.8814, -24.1528)
  line L1006 (24.8814, -23.6528) -> (22.3814, -23.6528)
  line L1007 (22.3814, -24.1528) -> (24.8814, -24.1528)
  line L1008 (258.1253, -5.1029) -> (255.6253, -5.1029)
  line L1009 (255.6253, -4.6029) -> (258.1253, -4.6029)
  line L1010 (260.6253, -5.1029) -> (260.6253, -4.6029)
  line L1011 (260.6253, -19.1022) -> (260.6253, -19.6022)
  line L1012 (258.1253, -19.1022) -> (260.6253, -19.1022)
  line L1013 (260.6253, -4.6029) -> (258.1253, -4.6029)
  line L1014 (255.6253, -5.1029) -> (255.6253, -4.6029)
  line L1015 (260.6253, -19.6022) -> (258.1253, -19.6022)
  line L1016 (258.1253, -19.1022) -> (255.6253, -19.1022)
  line L1017 (255.6253, -19.1022) -> (255.6253, -19.6022)
  line L1018 (258.1253, -5.1029) -> (260.6253, -5.1029)
  line L1019 (255.6253, -19.6022) -> (258.1253, -19.6022)
  line L1020 (224.7878, -19.1023) -> (222.2878, -19.1023)
  line L1021 (222.2878, -19.1023) -> (222.2878, -19.6023)
  line L1022 (222.2878, -19.6023) -> (224.7878, -19.6023)
  line L1023 (224.7878, -19.1023) -> (227.2878, -19.1023)
  line L1024 (227.2878, -19.1023) -> (227.2878, -19.6023)
  line L1025 (227.2878, -19.6023) -> (224.7878, -19.6023)
  line L1026 (224.7878, -5.1029) -> (227.2878, -5.1029)
  line L1027 (222.2878, -4.6029) -> (224.7878, -4.6029)
  line L1028 (222.2878, -5.1029) -> (222.2878, -4.6029)
  line L1029 (224.7878, -5.1029) -> (222.2878, -5.1029)
  line L1030 (227.2878, -5.1029) -> (227.2878, -4.6029)
  line L1031 (227.2878, -4.6029) -> (224.7878, -4.6029)
  line L1032 (250.9813, -38.1522) -> (248.4813, -38.1522)
  line L1033 (248.4813, -38.1522) -> (248.4813, -38.6522)
  line L1034 (248.4813, -38.6522) -> (250.9813, -38.6522)
  line L1035 (250.9813, -38.1522) -> (253.4813, -38.1522)
  line L1036 (253.4813, -38.1522) -> (253.4813, -38.6522)
  line L1037 (253.4813, -38.6522) -> (250.9813, -38.6522)
  line L1038 (250.9813, -24.1528) -> (248.4813, -24.1528)
  line L1039 (253.4813, -23.6528) -> (250.9813, -23.6528)
  line L1040 (253.4813, -24.1528) -> (253.4813, -23.6528)
  line L1041 (250.9813, -24.1528) -> (253.4813, -24.1528)
  line L1042 (248.4813, -24.1528) -> (248.4813, -23.6528)
  line L1043 (248.4813, -23.6528) -> (250.9813, -23.6528)
  line L1044 (143.8253, -19.1023) -> (141.3253, -19.1023)
  line L1045 (141.3253, -19.1023) -> (141.3253, -19.6023)
  line L1046 (141.3253, -19.6023) -> (143.8253, -19.6023)
  line L1047 (143.8253, -19.1023) -> (146.3253, -19.1023)
  line L1048 (146.3253, -19.1023) -> (146.3253, -19.6023)
  line L1049 (146.3253, -19.6023) -> (143.8253, -19.6023)
  line L1050 (143.8253, -5.1029) -> (146.3253, -5.1029)
  line L1051 (141.3253, -4.6029) -> (143.8253, -4.6029)
  line L1052 (141.3253, -5.1029) -> (141.3253, -4.6029)
  line L1053 (146.3253, -5.1029) -> (146.3253, -4.6029)
  line L1054 (143.8253, -5.1029) -> (141.3253, -5.1029)
  line L1055 (146.3253, -4.6029) -> (143.8253, -4.6029)
  line L1056 (62.8626, -19.1023) -> (60.3626, -19.1023)
  line L1057 (60.3626, -19.1023) -> (60.3626, -19.6023)
  line L1058 (60.3626, -19.6023) -> (62.8626, -19.6023)
  line L1059 (62.8626, -19.1023) -> (65.3626, -19.1023)
  line L1060 (65.3626, -19.1023) -> (65.3626, -19.6023)
  line L1061 (65.3626, -19.6023) -> (62.8626, -19.6023)
  line L1062 (15.2377, -19.1023) -> (12.7377, -19.1023)
  line L1063 (12.7377, -19.1023) -> (12.7377, -19.6023)
  line L1064 (12.7377, -19.6023) -> (15.2377, -19.6023)
  line L1065 (15.2377, -19.1023) -> (17.7377, -19.1023)
  line L1066 (17.7377, -19.1023) -> (17.7377, -19.6023)
  line L1067 (17.7377, -19.6023) -> (15.2377, -19.6023)
  line L1068 (65.3626, -4.6029) -> (62.8626, -4.6029)
  line L1069 (62.8626, -5.1029) -> (60.3626, -5.1029)
  line L1070 (60.3626, -4.6029) -> (62.8626, -4.6029)
  line L1071 (62.8626, -5.1029) -> (65.3626, -5.1029)
  line L1072 (65.3626, -5.1029) -> (65.3626, -4.6029)
  line L1073 (60.3626, -5.1029) -> (60.3626, -4.6029)
  line L1074 (15.2377, -5.1029) -> (12.7377, -5.1029)
  line L1075 (17.7377, -4.6029) -> (15.2377, -4.6029)
  line L1076 (12.7377, -5.1029) -> (12.7377, -4.6029)
  line L1077 (15.2377, -5.1029) -> (17.7377, -5.1029)
  line L1078 (17.7377, -5.1029) -> (17.7377, -4.6029)
  line L1079 (12.7377, -4.6029) -> (15.2377, -4.6029)
extrude "Extrude3" cut sketch "plate switch clips" against normal blind 2.5 contours L3 L925 L926 L927 L928 L931 L934 | L1 L924 L929 L930 L932 L933 L935 | L4 L474 L475 L476 L477 L478 L479 | L6 L468 L469 L470 L471 L472 L473 | L8 L486 L487 L488 L489 L490 L491 | L10 L576 L577 L578 L579 L580 L581 | L15 L552 L553 L554 L555 L556 L557 | L13 L642 L643 L644 L645 L646 L647 | L19 L841 L844 L847 L849 L850 L851 | L17 L840 L842 L843 L845 L846 L848 | L20 L937 L938 L939 L944 L946 L947 | L22 L936 L940 L941 L942 L943 L945 | L27 L960 L964 L965 L967 L969 L971 | L25 L961 L962 L963 L966 L968 L970 | L28 L901 L902 L905 L908 L909 L911 | L30 L900 L903 L904 L906 L907 L910 | L35 L618 L619 L620 L621 L622 L623 | L33 L528 L529 L530 L531 L532 L533 | L40 L408 L409 L410 L411 L412 L413 | L42 L414 L415 L416 L417 L418 L419 | L47 L672 L673 L674 L675 L676 L677 | L45 L678 L679 L680 L681 L682 L683 | L48 L1074 L1075 L1076 L1077 L1078 L1079 | L50 L1062 L1063 L1064 L1065 L1066 L1067 | L52 L624 L625 L626 L627 L628 L629 | L54 L534 L535 L536 L537 L538 L539 | L56 L360 L361 L362 L363 L364 L365 | L58 L366 L367 L368 L369 L370 L371 | L63 L654 L655 L656 L657 L658 L659 | L61 L564 L565 L566 L567 L568 L569 | L64 L865 L867 L869 L872 L873 L875 | L66 L864 L866 L868 L870 L871 L874 | L71 L734 L735 L737 L739 L742 L743 | L69 L732 L733 L736 L738 L740 L741 | L75 L348 L350 L353 L354 L355 L359 | L73 L349 L351 L352 L356 L357 L358 | L76 L852 L854 L855 L857 L858 L862 | L78 L853 L856 L859 L860 L861 L863 | L83 L480 L481 L482 L483 L484 L485 | L81 L570 L571 L572 L573 L574 L575 | L87 L794 L797 L798 L799 L800 L802 | L85 L792 L793 L795 L796 L801 L803 | L88 L708 L711 L712 L715 L716 L719 | L90 L709 L710 L713 L714 L717 L718 | L96 L973 L974 L975 L976 L977 L982 | L98 L972 L978 L979 L980 L981 L983 | L103 L300 L301 L302 L303 L304 L305 | L101 L306 L307 L308 L309 L310 L311 | L107 L996 L997 L998 L999 L1000 L1001 | L105 L1002 L1003 L1004 L1005 L1006 L1007 | L108 L985 L987 L988 L990 L991 L992 | L110 L984 L986 L989 L993 L994 L995 | L119 L804 L805 L806 L808 L814 L815 | L117 L807 L809 L810 L811 L812 L813 | L123 L780 L781 L784 L785 L786 L790 | L121 L782 L783 L787 L788 L789 L791 | L124 L648 L649 L650 L651 L652 L653 | L126 L558 L559 L560 L561 L562 L563 | L132 L594 L595 L596 L597 L598 L599 | L134 L504 L505 L506 L507 L508 L509 | L136 L889 L890 L892 L894 L896 L897 | L138 L888 L891 L893 L895 L898 L899 | L143 L606 L607 L608 L609 L610 L611 | L141 L516 L517 L518 L519 L520 L521 | L147 L768 L769 L774 L775 L776 L778 | L145 L770 L771 L772 L773 L777 L779 | L148 L450 L451 L452 L453 L454 L455 | L150 L444 L445 L446 L447 L448 L449 | L155 L318 L319 L320 L321 L322 L323 | L153 L312 L313 L314 L315 L316 L317 | L156 L432 L433 L434 L435 L436 L437 | L158 L438 L439 L440 L441 L442 L443 | L166 L1026 L1027 L1028 L1029 L1030 L1031 | L168 L1020 L1021 L1022 L1023 L1024 L1025 | L170 L582 L583 L584 L585 L586 L587 | L172 L492 L493 L494 L495 L496 L497 | L177 L384 L385 L386 L387 L388 L389 | L175 L390 L391 L392 L393 L394 L395 | L181 L948 L949 L950 L951 L955 L956 | L179 L952 L953 L954 L957 L958 L959 | L185 L720 L723 L724 L727 L729 L730 | L183 L721 L722 L725 L726 L728 L731 | L186 L698 L699 L700 L703 L706 L707 | L188 L696 L697 L701 L702 L704 L705 | L190 L546 L547 L548 L549 L550 L551 | L192 L636 L637 L638 L639 L640 L641 | L197 L1038 L1039 L1040 L1041 L1042 L1043 | L195 L1032 L1033 L1034 L1035 L1036 L1037 | L198 L759 L760 L762 L765 L766 L767 | L200 L756 L757 L758 L761 L763 L764 | L202 L600 L601 L602 L603 L604 L605 | L204 L510 L511 L512 L513 L514 L515 | L209 L1068 L1069 L1070 L1071 L1072 L1073 | L207 L1056 L1057 L1058 L1059 L1060 L1061 | L213 L1008 L1009 L1010 L1013 L1014 L1018 | L211 L1011 L1012 L1015 L1016 L1017 L1019 | L218 L456 L457 L458 L459 L460 L461 | L220 L462 L463 L464 L465 L466 L467 | L225 L612 L613 L614 L615 L616 L617 | L223 L522 L523 L524 L525 L526 L527 | L226 L912 L913 L914 L915 L919 L920 | L228 L916 L917 L918 L921 L922 L923 | L236 L396 L397 L398 L399 L400 L401 | L238 L402 L403 L404 L405 L406 L407 | L240 L540 L541 L542 L543 L544 L545 | L242 L630 L631 L632 L633 L634 L635 | L248 L684 L685 L686 L687 L688 L689 | L250 L690 L691 L692 L693 L694 L695 | L252 L1044 L1045 L1046 L1047 L1048 L1049 | L254 L1050 L1051 L1052 L1053 L1054 L1055 | L256 L660 L661 L662 L663 L664 L665 | L258 L666 L667 L668 L669 L670 L671 | L263 L876 L877 L878 L879 L880 L881 | L261 L882 L883 L884 L885 L886 L887 | L267 L337 L339 L340 L344 L345 L346 | L265 L336 L338 L341 L342 L343 L347 | L268 L816 L817 L818 L819 L820 L821 | L270 L822 L823 L824 L825 L826 L827 | L275 L327 L329 L330 L333 L334 L335 | L273 L324 L325 L326 L328 L331 L332 | L279 L744 L746 L747 L753 L754 L755 | L277 L745 L748 L749 L750 L751 L752 | L280 L498 L499 L500 L501 L502 L503 | L282 L588 L589 L590 L591 L592 L593 | L284 L378 L379 L380 L381 L382 L383 | L286 L372 L373 L374 L375 L376 L377 | L291 L426 L427 L428 L429 L430 L431 | L289 L420 L421 L422 L423 L424 L425 | L295 L833 L834 L835 L836 L837 L839 | L293 L828 L829 L830 L831 L832 L838 bodies 1
sketch "Right Side Profile" plane through (312.1758, 0, 0) normal (1, 0, 0) x (0, 0, -1)
  line L0 (-3.8481, 7) -> (-3.8481, -4)
  line L1 (-3.8481, -4) -> (104.2517, -4)
  line L2 (104.2517, -4) -> (104.2517, 7)
  line L3 (104.2517, 7) -> (-3.8481, 7)
  line L4 (104.2517, 0) -> (-3.8481, 0)
  line L5 (-3.8481, -4) -> (104.2517, -4)
  line L6 (-3.8481, -4) -> (-3.8481, -10)
  line L7 (104.2517, -4) -> (104.2517, -12)
  line L8 (104.2517, -12) -> (19.012, -12)
  line L9 (104.2517, -12) -> (96.2034, -18.7534)
  line L10 (96.2034, -18.7534) -> (-3.8481, -10)
extrude "Extrude9" add sketch "Right Side Profile" against normal blind 317.65 separate body contours L1 L5 L6 L7 L8 L10 | L8 L9 L10 makes body 2